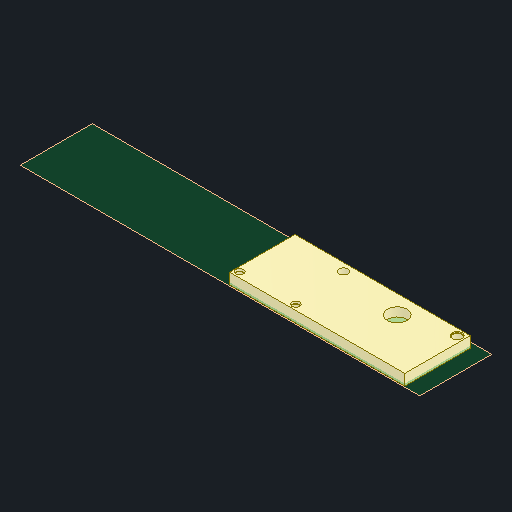
# Autodesk Inventor part: right_gear_holder
Saved by Autodesk Inventor 2023 (Build 270158000, 158)
## iProperties
Created: 2024-04-30
Part Number: right_gear_holder
Material: Nylon 6/6
Document SubType Name: Modeling
Designer: szymo
Density: 1.13 g/cm^3
Appearance: Nylon 6
Mass: 13.1533 g
Surface Area: 62.1133 cm^2
Volume: 11.6401 cm^3
Author: szymo
Autodesk Inventor part; units mm, degrees
ref_plane "YZ Plane" through (0, 0, 0) normal (1, 0, 0) x (0, 1, 0)
ref_plane "XZ Plane" through (0, 0, 0) normal (0, 1, 0) x (-1, 0, 0)
ref_plane "XY Plane" through (0, 0, 0) normal (0, 0, 1) x (1, 0, 0)
ref_plane "Work Plane3" through (-75.5, 11, 0) normal (0, -1, 0) x (1, 0, 0)
sketch "Sketch3" plane through (-75.5, 11, 0) normal (0, -1, 0) x (1, 0, 0)
  line L0 (86.15, 30) -> (166.5, 30) projected
  line L1 (166.5, 0) -> (166.5, 30) projected
  line L2 (116.5, 0) -> (166.5, 0) projected
  line L3 (86.15, 30) -> (86.15, 14.5) projected
  line L4 (86.15, 30) -> (166.5, 30)
  line L5 (166.5, 30) -> (166.5, 0)
  line L6 (166.5, 0) -> (86.15, 0)
  line L7 (86.15, 0) -> (86.15, 30)
  point P0 (75.5, 0)
  constraints: 8 end point, 2 parallel, 1 horizontal, 1 perpendicular
extrude "Extrusion1" add sketch "Sketch3" along normal blind 1
sketch "Sketch4" plane through (-75.5, 11, 0) normal (0, 1, 0) x (1, 0, 0)
  line L0 (86.15, 0) -> (166.5, 0) projected
  line L1 (86.15, -30) -> (86.15, 0) projected
  line L2 (166.5, -30) -> (86.15, -30) projected
  line L3 (166.5, 0) -> (166.5, -30) projected
  circle A0 centre (141.5, -8.5) radius 4.5 projected
  circle A1 centre (111.9101, -3.5563) radius 2 projected
  circle A2 centre (111.9101, -3.5563) radius 6
  line L4 (117.9101, -3.5563) -> (117.9101, 0)
  line L5 (86.15, 0) -> (166.5, 0) projected
  line L6 (105.9101, -3.5563) -> (105.9101, 0)
  point P0 (75.5, 0)
  point P1 (107.0777, 0)
  dimension "d2" = 12
  constraints: 4 end point, 2 point on circle, 2 point on line, 1 centre point, 1 coincident, 1 parallel, 1 perpendicular, 1 tangent
  measures "d2" diameter of A2
extrude "Extrusion2" add sketch "Sketch4" along normal blind 1 contours L0 A2 L6 | L0 A2 | L0 L4 A2 | A1 picked at (111.8297, -0.5236)
sketch "Sketch5" plane through (-75.5, 12, 0) normal (0, 1, 0) x (1, 0, 0)
  line L0 (117.9101, 0) -> (105.9101, 0) projected
  line L1 (105.9101, 0) -> (105.9101, -3.5563) projected
  arc A0 (105.9101, -3.5563) -> (117.9101, -3.5563) centre (111.9101, -3.5563) ccw projected
  line L2 (117.9101, -3.5563) -> (117.9101, 0) projected
  circle A1 centre (111.9101, -3.5563) radius 2 projected
  point P0 (75.5, 0)
extrude "Extrusion3" add sketch "Sketch5" along normal blind 3
sketch "Sketch6" plane through (-75.5, 11, 0) normal (0, 1, 0) x (1, 0, 0)
  circle A0 centre (141.5, -8.5) radius 4.5 projected
  circle A1 centre (141.5, -8.5) radius 8.5
  line L0 (150, -8.5) -> (149.6698, 0)
  line L1 (86.15, 0) -> (166.5, 0) projected
  line L2 (133, -8.5) -> (133, 0)
  line L3 (117.9101, 0) -> (166.5, 0) projected
  point P0 (75.5, 0)
  dimension "d7" = 17
  constraints: 4 end point, 2 point on circle, 2 point on line, 1 centre point, 1 coincident, 1 vertical
  measures "d7" diameter of A1
ref_plane "Work Plane4" through (60.3074, 16, 2.8074) normal (0, -1, 0) x (0.988717, 0, 0.1497953)
extrude "Extrusion4" add sketch "Sketch6" along normal blind 4 contours A1 L0 | L2 L1 A1 | L1 L0 A1 picked at (148.4648, -7.0125)
sketch "Sketch7" plane through (-75.5, 11, 0) normal (0, 1, 0) x (1, 0, 0)
  line L0 (166.5, -30) -> (86.15, -30) projected
  line L1 (166.5, 0) -> (166.5, -30) projected
  line L2 (86.15, -30) -> (86.15, 0) projected
  line L3 (86.15, 0) -> (105.9101, 0) projected
  line L4 (105.9101, 0) -> (105.9101, -3.5563) projected
  arc A0 (105.9101, -3.5563) -> (117.9101, -3.5563) centre (111.9101, -3.5563) ccw projected
  line L5 (117.9101, -3.5563) -> (117.9101, 0) projected
  line L6 (117.9101, 0) -> (105.9101, 0) projected
  circle A1 centre (111.9101, -3.5563) radius 2 projected
  line L7 (149.6698, 0) -> (133, 0) projected
  line L8 (133, 0) -> (133, -8.5) projected
  arc A2 (133, -8.5) -> (150, -8.5) centre (141.5, -8.5) ccw projected
  line L9 (150, -8.5) -> (149.6698, 0) projected
  circle A3 centre (141.5, -8.5) radius 4.5 projected
  line L10 (149.6698, 0) -> (166.5, 0) projected
  line L11 (117.9101, 0) -> (133, 0) projected
  point P0 (75.5, 0)
extrude "Extrusion5" add sketch "Sketch7" along normal blind 4 contours L0 L2 L3 L4 A0 L5 L11 L8 A2 L9 L10 L1
sketch "Sketch8" plane through (-75.5, 15, 0) normal (0, 1, 0) x (1, 0, 0)
  circle A0 centre (114, -27.5) radius 1.55 projected
  circle A1 centre (88.25, -27.5) radius 1.55 projected
  point P0 (75.5, 0)
  constraints: 2 coincident
hole "Hole1" at (12.75, 15, 27.5) at (38.5, 15, 27.5) direction (0, -1, 0) diameter 3 depth 4 counterbore diameter 3.5 counterbore depth 1
sketch "Sketch9" plane through (-75.5, 15, 0) normal (0, 1, 0) x (1, 0, 0)
  circle A0 centre (163.5, -3) radius 1.8 projected
  point P0 (75.5, 0)
hole "Hole2" at (88, 15, 3) direction (0, -1, 0) diameter 4 depth 4.5 counterbore diameter 4.6 counterbore depth 0.5
body "Solid1"
